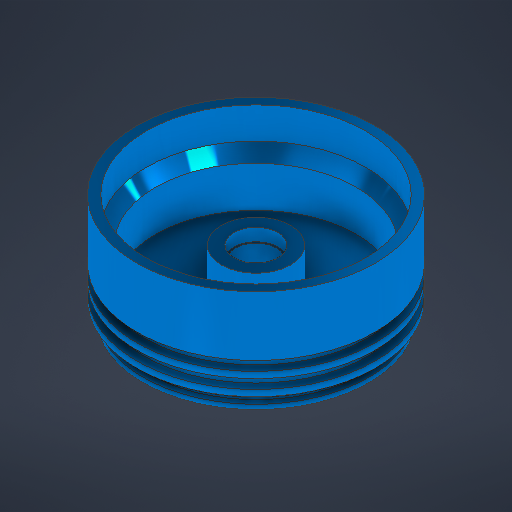
# Autodesk Inventor part: PARTE_SUPERIOR_IGNICION
Saved by Autodesk Inventor 2025 (Build 290162010, 162A)
## iProperties
Created: 2024-07-24
Part Number: PARTE_SUPERIOR_IGNICION
Material: Genérico
Document SubType Name: Modeling
Designer: hansm
Density: 1 g/cm^3
Appearance: Valor por defecto
Author: hansm
Autodesk Inventor part; units mm, degrees
ref_plane "YZ Plane" through (0, 0, 0) normal (1, 0, 0) x (0, 1, 0)
ref_plane "XZ Plane" through (0, 0, 0) normal (0, 1, 0) x (-1, 0, 0)
ref_plane "XY Plane" through (0, 0, 0) normal (0, 0, 1) x (1, 0, 0)
sketch "Boceto2" plane through (0, 0, 0) normal (0, 0, 1) x (1, 0, 0)
  line L0 (-6, 9) -> (-6.5, 10)
  line L1 (-6.5, 10) -> (-6.5, 16)
  line L2 (-6.5, 16) -> (-7, 16)
  line L3 (-7, 16) -> (-7, 20)
  line L4 (-7, 20) -> (-11, 20)
  line L5 (-11, 20) -> (-11, 7)
  line L6 (-11, 7) -> (-32, 7)
  line L7 (-32, 7) -> (-32, 20)
  line L8 (-32, 20) -> (-35, 24)
  line L9 (-35, 34) -> (-38, 34)
  line L10 (-38, 34) -> (-38, 15)
  line L11 (-38, 15) -> (-35.5, 15)
  line L12 (-35.5, 12) -> (-38, 12)
  line L13 (-38, 10) -> (-35.5, 10)
  line L14 (-35.5, 7) -> (-38, 7)
  line L15 (-38, 5) -> (-36, 5)
  line L16 (-36, 5) -> (-36, 3.5)
  line L17 (-36, 3.5) -> (-34.2, 3.5)
  line L18 (-34.2, 3.5) -> (-34.2, 1.5)
  line L19 (-34.2, 1.5) -> (-36, 1.5)
  line L20 (-36, 1.5) -> (-36, 0)
  line L21 (-6, 9) -> (-6, 0)
  line L22 (-36, 0) -> (-6, 0)
  line L23 (-35.5, 10) -> (-35.5, 7)
  line L24 (-38, 12) -> (-38, 10)
  line L25 (-35, 34) -> (-35, 24)
  line L26 (-35.5, 15) -> (-35.5, 12)
  line L27 (0, -6.8) -> (0, 40.8) projected
  line L28 (-38, 7) -> (-38, 5)
  point P0 (0, 0)
  dimension "d2" = 9
  dimension "d3" = 1
  dimension "d4" = 0.5
  dimension "d5" = 0.5
  dimension "d6" = 6
  dimension "d7" = 4
  dimension "d8" = 4
  dimension "d9" = 7
  dimension "d16" = 1.5
  dimension "d17" = 1.8
  dimension "d19" = 2
  dimension "d20" = 1.5
  dimension "d21" = 2
  dimension "d23" = 3
  dimension "d24" = 2
  dimension "d25" = 3
  dimension "d33" = 38
  dimension "d35" = 6
  dimension "d38" = 4
  dimension "d39" = 21
  dimension "d40" = 13
  dimension "d42" = 2.5
  dimension "d43" = 3
  dimension "d44" = 2.5
  dimension "d49" = 2
  dimension "d51" = 10
  constraints: 56 end point, 13 perpendicular, 6 vertical, 2 horizontal, 1 collinear, 1 point on line
  measures "d2" distance of L0.start L21.end
  measures "d3" vertical distance of L0.end L0.start
  measures "d4" horizontal distance of L0.start L0.end
  measures "d5" distance of L1.end L2.end
  measures "d6" distance of L0.end L1.end
  measures "d7" distance of L2.end L3.end
  measures "d8" distance of L3.end L4.end
  measures "d9" distance from line of L22 L5.end
  measures "d16" distance of L19.end L20.end
  measures "d17" distance of L18.end L19.end
  measures "d19" distance of L17.end L18.end
  measures "d20" distance of L15.end L16.end
  measures "d21" distance of L14.end L15.start
  measures "d23" distance of L13.end L14.start
  measures "d24" distance of L12.end L13.start
  measures "d25" distance of L11.end L12.start
  measures "d33" horizontal distance of point (0, 0) L9.end
  measures "d35" distance of point (0, 0) L21.end
  measures "d38" vertical distance of L7.end L8.end
  measures "d39" distance of L5.end L6.end
  measures "d40" distance of L6.end L7.end
  measures "d42" distance of L10.end L11.end
  measures "d43" distance of L9.start L9.end
  measures "d44" distance of L13.start L13.end
  measures "d49" distance of L15.start L15.end
  measures "d51" distance of L9.start L8.end
revolve "Revolución1" add sketch "Boceto2" angle 360 about axis through (0, -10, 0) along (0, 1, 0)
sketch "Boceto3" plane through (0, 7, 0) normal (0, 1, 0) x (1, 0, 0)
  line L0 (-0.0776, -21.9999) -> (-19.0136, 11.0671) construction
  line L1 (-19.0136, 11.0671) -> (19.0912, 10.9327) construction
  line L2 (19.0912, 10.9327) -> (-0.0776, -21.9999) construction
  circle A0 centre (0, 0) radius 11 construction
  circle A1 centre (0, 0) radius 11 projected
  circle A2 centre (-0.0776, -21.9999) radius 2.5
  circle A3 centre (19.0912, 10.9327) radius 2.5
  circle A4 centre (-19.0136, 11.0671) radius 2.5
  dimension "d56" = 5
  constraints: 6 end point, 5 coincident, 4 centre point, 2 equal radius, 1 tangent, 7 other
  measures "d56" diameter of A2
extrude "Extrusión1" cut sketch "Boceto3" against normal up to surface (7 mm away) contours A2 | A3 | A4
